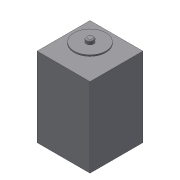
# Autodesk Inventor part: Wind Trubin Engine
Saved by Autodesk Inventor 2015 SP1 (Build 190203100, 203)
## iProperties
Created: 2015-08-24
Part Number: Wind Trubin Engine
Material: 一般
Document SubType Name: Modeling
Designer: nobuhiro
Density: 1 g/cm^3
Appearance: 既定
Author: nobuhiro
Autodesk Inventor part; units mm, degrees
ref_plane "YZ Plane" through (0, 0, 0) normal (1, 0, 0) x (0, 1, 0)
ref_plane "XZ Plane" through (0, 0, 0) normal (0, 1, 0) x (-1, 0, 0)
ref_plane "XY Plane" through (0, 0, 0) normal (0, 0, 1) x (1, 0, 0)
sketch "スケッチ1" plane through (0, 0, 0) normal (0, 0, 1) x (1, 0, 0)
  line L0 (-100, -100) -> (100, -100)
  line L1 (100, -100) -> (100, 100)
  line L2 (100, 100) -> (-100, 100)
  line L3 (-100, 100) -> (-100, -100)
  line L4 (-100, -100) -> (100, 100) construction
  line L5 (100, -100) -> (-100, 100) construction
  point P0 (0, 0)
  dimension "d0" = 200
  constraints: 12 end point, 2 midpoint, 2 parallel, 2 perpendicular, 1 horizontal
  measures "d0" distance of L2.end L0.start
extrude "押し出し1" add sketch "スケッチ1" along normal blind 300
sketch "スケッチ2" plane through (0, 0, 0) normal (1, 0, 0) x (0, 1, 0)
  line L0 (0, 300) -> (14, 300)
  line L1 (14, 300) -> (14, 340)
  line L2 (9, 345) -> (0, 345)
  line L3 (0, 345) -> (0, 300)
  line L4 (100, 300) -> (-100, 300) projected
  line L5 (0, 330) -> (60, 330)
  line L6 (60, 330) -> (60, 325)
  line L7 (60, 325) -> (0, 325)
  line L8 (0, 325) -> (0, 330)
  arc A0 (14, 340) -> (9, 345) centre (9, 340) ccw
  point P0 (0, 0)
  dimension "d3" = 14
  dimension "d4" = 45
  dimension "d5" = 5
  dimension "d6" = 60
  dimension "d7" = 15
  dimension "d8" = 5
  dimension "d10" = 25
  constraints: 16 end point, 4 parallel, 2 horizontal, 2 perpendicular, 2 point on circle, 2 tangent, 1 centre point, 1 collinear, 1 point on line, 1 vertical alignment
  measures "d3" distance between parallel lines of L1 L3
  measures "d4" distance of L2.end L0.start
  measures "d5" distance of L5.end L6.end
  measures "d6" distance between parallel lines of L3 L6
  measures "d7" distance between parallel lines of L2 L5
  measures "d8" radius of A0
  measures "d10" distance between parallel lines of L4 L7
revolve "回転1" add sketch "スケッチ2" angle 360 about axis through (0, 0, 345) along (0, 0, -1)
